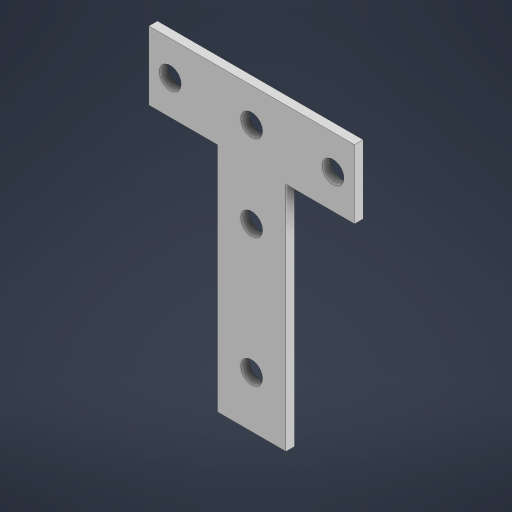
# Autodesk Inventor part: T-shaped_plate
Saved by Autodesk Inventor 2024 (Build 280153000, 153)
## iProperties
Created: 2023-04-15
Part Number: T-shaped_plate
Material: Типовые
Document SubType Name: Modeling
Designer: user
Density: 1 g/cm^3
Appearance: По умолчанию
Author: user
Autodesk Inventor part; units mm, degrees
ref_plane "YZ Plane" through (0, 0, 0) normal (1, 0, 0) x (0, 1, 0)
ref_plane "XZ Plane" through (0, 0, 0) normal (0, 1, 0) x (-1, 0, 0)
ref_plane "XY Plane" through (0, 0, 0) normal (0, 0, 1) x (1, 0, 0)
sketch "Эскиз1" plane through (0, 0, 0) normal (0, 0, 1) x (1, 0, 0)
  line L0 (0, 0) -> (0, 54)
  line L1 (0, 54) -> (-16, 54)
  line L2 (-16, 54) -> (-16, 70)
  line L3 (-16, 70) -> (32, 70)
  line L4 (32, 70) -> (32, 54)
  line L5 (32, 54) -> (16, 54)
  line L6 (16, 54) -> (16, 0)
  line L7 (16, 0) -> (0, 0)
  circle A0 centre (-11, 62) radius 2.55
  circle A1 centre (8, 62) radius 2.55
  circle A2 centre (27, 62) radius 2.55
  circle A3 centre (8, 42) radius 2.55
  circle A4 centre (8, 12) radius 2.55
  point P0 (-8, 54)
  point P1 (24, 54)
  point P2 (8, 70)
  point P3 (-16, 62)
  dimension "d0" = 16
  dimension "d1" = 70
  dimension "d2" = 16
  dimension "d3" = 48
  dimension "d4" = 5
  dimension "d5" = 5
  dimension "d6" = 5.1
  dimension "d7" = 20
  dimension "d8" = 30
  constraints: 16 end point, 6 perpendicular, 5 centre point, 4 equal radius, 4 horizontal alignment, 4 midpoint, 3 vertical alignment, 1 collinear, 1 horizontal, 1 vertical
  measures "d0" distance of L6.end L0.start
  measures "d1" vertical distance of L2.end L0.start
  measures "d2" distance of L3.end L4.end
  measures "d3" distance of L2.end L3.end
  measures "d4" horizontal distance of L3.end A2.centre
  measures "d5" horizontal distance of L2.end A0.centre
  measures "d6" diameter of A2
  measures "d7" distance of A3.centre A1.centre
  measures "d8" distance of A4.centre A3.centre
extrude "Выдавливание1" add sketch "Эскиз1" along normal blind 2
